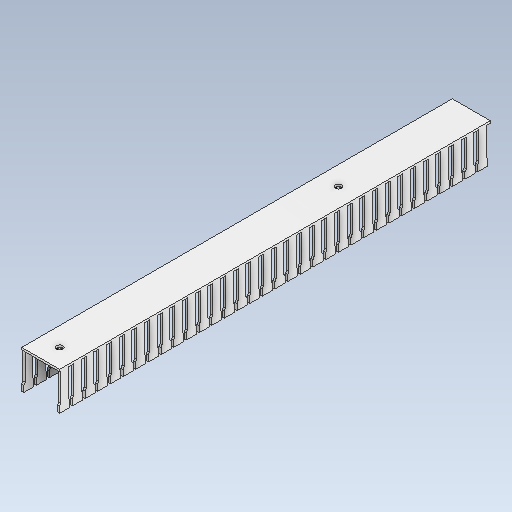
# Autodesk Inventor part: Pasabable Ranurado 30 x 30 L = 430
Saved by Autodesk Inventor 2020 (Build 240168000, 168)
## iProperties
Created: 2020-07-02
Part Number: Pasabable Ranurado 30 x 30 L = 430
Material: PVC-Piping
Document SubType Name: Modeling
Designer: Hernan
Density: 1.4 g/cm^3
Appearance: Smooth - White
Author: Hernan
Autodesk Inventor part; units mm, degrees
ref_plane "YZ Plane" through (0, 0, 0) normal (1, 0, 0) x (0, 1, 0)
ref_plane "XZ Plane" through (0, 0, 0) normal (0, 1, 0) x (-1, 0, 0)
ref_plane "XY Plane" through (0, 0, 0) normal (0, 0, 1) x (1, 0, 0)
sketch "Sketch1" plane through (0, 0, 0) normal (0, 0, 1) x (1, 0, 0)
  line L0 (-26.9918, -9.5406) -> (3.0082, -9.5406)
  line L1 (3.0082, -9.5406) -> (3.0082, 20.4594)
  line L2 (3.0082, 20.4594) -> (-26.9918, 20.4594)
  line L3 (-26.9918, 20.4594) -> (-26.9918, -9.5406)
  line L4 (1.3082, 20.4594) -> (1.3082, -9.5406)
  line L5 (-26.9918, -7.8406) -> (3.0082, -7.8406)
  line L6 (-25.2918, 20.4594) -> (-25.2918, -9.5406)
  line L7 (-26.9918, 18.7594) -> (3.0082, 18.7594)
  point P0 (0, 0)
  point P1 (1.3082, 18.7594)
  point P2 (-25.2918, 18.7594)
  point P3 (-25.2918, -7.8406)
  point P4 (1.3082, -7.8406)
  dimension "d0" = 30
  dimension "d1" = 30
  dimension "d4" = 1.7
  dimension "d5" = 1.7
  dimension "d6" = 1.7
  dimension "d7" = 1.7
  constraints: 16 end point, 8 point on line, 3 horizontal, 3 perpendicular, 2 vertical
  measures "d0" distance of L0.start L0.end
  measures "d1" distance of L0.end L1.end
  measures "d4" distance between parallel lines of L2 L7
  measures "d5" distance between parallel lines of L3 L6
  measures "d6" distance between parallel lines of L0 L5
  measures "d7" distance between parallel lines of L1 L4
extrude "Extrusion1" add sketch "Sketch1" against normal blind 340
extrude "Extrusion2" cut sketch "Sketch1" against normal blind 380 contours L6 L5 L4 L0 | L6 L7 L4 L5
sketch "Boceto2" plane through (-26.9918, 20.4594, 0) normal (0, 1, 0) x (1, 0, 0)
  line L0 (0, 340) -> (30, 340) projected
  line L1 (30, 0) -> (0, 0) projected
  point P0 (26.9918, 0)
sketch "Boceto3" plane through (-26.9918, 20.4594, 0) normal (0, 1, 0) x (1, 0, 0)
  line L0 (28.3, 340) -> (1.7, 340) projected
  line L1 (30, 0) -> (0, 0) projected
  circle A0 centre (15, 235) radius 2.5
  circle A1 centre (15, 15) radius 2.5
  point P0 (26.9918, 0)
  dimension "d17" = 5
  dimension "d18" = 5
  dimension "d95" = 220
  dimension "d97" = 15
  constraints: 2 centre point
  measures "d17" diameter of A0
  measures "d18" diameter of A1
  measures "d95" distance of A1.centre A0.centre
  measures "d97" distance from line of L1 A1.centre
extrude "Extrusión3" cut sketch "Boceto3" against normal blind 10
sketch "Boceto4" plane through (-26.9918, -9.5406, 0) normal (-1, 0, 0) x (0, 0, 1)
  line L0 (0, 0) -> (-8, 0)
  line L1 (0, 0) -> (-340, 0) projected
  line L2 (-8, 0) -> (-8, 5)
  line L3 (-7, 6.5) -> (-7, 28.3)
  line L4 (0, 28.3) -> (-340, 28.3) projected
  line L5 (0, 30) -> (0, 0) projected
  line L6 (0, 0) -> (0, 5)
  line L7 (-1, 6.5) -> (-1, 28.3)
  line L8 (-8, 5) -> (-7, 6.5)
  line L9 (-1, 6.5) -> (0, 5)
  line L10 (-10, 0) -> (-18, 0)
  line L11 (-18, 0) -> (-18, 5)
  line L12 (-17, 6.5) -> (-17, 28.3)
  line L13 (-10, 0) -> (-10, 5)
  line L14 (-11, 6.5) -> (-11, 28.3)
  line L15 (-18, 5) -> (-17, 6.5)
  line L16 (-11, 6.5) -> (-10, 5)
  line L17 (-20, 0) -> (-28, 0)
  line L18 (-28, 0) -> (-28, 5)
  line L19 (-27, 6.5) -> (-27, 28.3)
  line L20 (-20, 0) -> (-20, 5)
  line L21 (-21, 6.5) -> (-21, 28.3)
  line L22 (-28, 5) -> (-27, 6.5)
  line L23 (-21, 6.5) -> (-20, 5)
  line L24 (-30, 0) -> (-38, 0)
  line L25 (-38, 0) -> (-38, 5)
  line L26 (-37, 6.5) -> (-37, 28.3)
  line L27 (-30, 0) -> (-30, 5)
  line L28 (-31, 6.5) -> (-31, 28.3)
  line L29 (-38, 5) -> (-37, 6.5)
  line L30 (-31, 6.5) -> (-30, 5)
  line L31 (-40, 0) -> (-48, 0)
  line L32 (-48, 0) -> (-48, 5)
  line L33 (-47, 6.5) -> (-47, 28.3)
  line L34 (-40, 0) -> (-40, 5)
  line L35 (-41, 6.5) -> (-41, 28.3)
  line L36 (-48, 5) -> (-47, 6.5)
  line L37 (-41, 6.5) -> (-40, 5)
  line L38 (-50, 0) -> (-58, 0)
  line L39 (-58, 0) -> (-58, 5)
  line L40 (-57, 6.5) -> (-57, 28.3)
  line L41 (-50, 0) -> (-50, 5)
  line L42 (-51, 6.5) -> (-51, 28.3)
  line L43 (-58, 5) -> (-57, 6.5)
  line L44 (-51, 6.5) -> (-50, 5)
  line L45 (-60, 0) -> (-68, 0)
  line L46 (-68, 0) -> (-68, 5)
  line L47 (-67, 6.5) -> (-67, 28.3)
  line L48 (-60, 0) -> (-60, 5)
  line L49 (-61, 6.5) -> (-61, 28.3)
  line L50 (-68, 5) -> (-67, 6.5)
  line L51 (-61, 6.5) -> (-60, 5)
  line L52 (-70, 0) -> (-78, 0)
  line L53 (-78, 0) -> (-78, 5)
  line L54 (-77, 6.5) -> (-77, 28.3)
  line L55 (-70, 0) -> (-70, 5)
  line L56 (-71, 6.5) -> (-71, 28.3)
  line L57 (-78, 5) -> (-77, 6.5)
  line L58 (-71, 6.5) -> (-70, 5)
  line L59 (-80, 0) -> (-88, 0)
  line L60 (-88, 0) -> (-88, 5)
  line L61 (-87, 6.5) -> (-87, 28.3)
  line L62 (-80, 0) -> (-80, 5)
  line L63 (-81, 6.5) -> (-81, 28.3)
  line L64 (-88, 5) -> (-87, 6.5)
  line L65 (-81, 6.5) -> (-80, 5)
  line L66 (-90, 0) -> (-98, 0)
  line L67 (-98, 0) -> (-98, 5)
  line L68 (-97, 6.5) -> (-97, 28.3)
  line L69 (-90, 0) -> (-90, 5)
  line L70 (-91, 6.5) -> (-91, 28.3)
  line L71 (-98, 5) -> (-97, 6.5)
  line L72 (-91, 6.5) -> (-90, 5)
  line L73 (-100, 0) -> (-108, 0)
  line L74 (-108, 0) -> (-108, 5)
  line L75 (-107, 6.5) -> (-107, 28.3)
  line L76 (-100, 0) -> (-100, 5)
  line L77 (-101, 6.5) -> (-101, 28.3)
  line L78 (-108, 5) -> (-107, 6.5)
  line L79 (-101, 6.5) -> (-100, 5)
  line L80 (-110, 0) -> (-118, 0)
  line L81 (-118, 0) -> (-118, 5)
  line L82 (-117, 6.5) -> (-117, 28.3)
  line L83 (-110, 0) -> (-110, 5)
  line L84 (-111, 6.5) -> (-111, 28.3)
  line L85 (-118, 5) -> (-117, 6.5)
  line L86 (-111, 6.5) -> (-110, 5)
  line L87 (-120, 0) -> (-128, 0)
  line L88 (-128, 0) -> (-128, 5)
  line L89 (-127, 6.5) -> (-127, 28.3)
  line L90 (-120, 0) -> (-120, 5)
  line L91 (-121, 6.5) -> (-121, 28.3)
  line L92 (-128, 5) -> (-127, 6.5)
  line L93 (-121, 6.5) -> (-120, 5)
  line L94 (-130, 0) -> (-138, 0)
  line L95 (-138, 0) -> (-138, 5)
  line L96 (-137, 6.5) -> (-137, 28.3)
  line L97 (-130, 0) -> (-130, 5)
  line L98 (-131, 6.5) -> (-131, 28.3)
  line L99 (-138, 5) -> (-137, 6.5)
  line L100 (-131, 6.5) -> (-130, 5)
  line L101 (-140, 0) -> (-148, 0)
  line L102 (-148, 0) -> (-148, 5)
  line L103 (-147, 6.5) -> (-147, 28.3)
  line L104 (-140, 0) -> (-140, 5)
  line L105 (-141, 6.5) -> (-141, 28.3)
  line L106 (-148, 5) -> (-147, 6.5)
  line L107 (-141, 6.5) -> (-140, 5)
  line L108 (-150, 0) -> (-158, 0)
  line L109 (-158, 0) -> (-158, 5)
  line L110 (-157, 6.5) -> (-157, 28.3)
  line L111 (-150, 0) -> (-150, 5)
  line L112 (-151, 6.5) -> (-151, 28.3)
  line L113 (-158, 5) -> (-157, 6.5)
  line L114 (-151, 6.5) -> (-150, 5)
  line L115 (-160, 0) -> (-168, 0)
  line L116 (-168, 0) -> (-168, 5)
  line L117 (-167, 6.5) -> (-167, 28.3)
  line L118 (-160, 0) -> (-160, 5)
  line L119 (-161, 6.5) -> (-161, 28.3)
  line L120 (-168, 5) -> (-167, 6.5)
  line L121 (-161, 6.5) -> (-160, 5)
  line L122 (-170, 0) -> (-178, 0)
  line L123 (-178, 0) -> (-178, 5)
  line L124 (-177, 6.5) -> (-177, 28.3)
  line L125 (-170, 0) -> (-170, 5)
  line L126 (-171, 6.5) -> (-171, 28.3)
  line L127 (-178, 5) -> (-177, 6.5)
  line L128 (-171, 6.5) -> (-170, 5)
  line L129 (-180, 0) -> (-188, 0)
  line L130 (-188, 0) -> (-188, 5)
  line L131 (-187, 6.5) -> (-187, 28.3)
  line L132 (-180, 0) -> (-180, 5)
  line L133 (-181, 6.5) -> (-181, 28.3)
  line L134 (-188, 5) -> (-187, 6.5)
  line L135 (-181, 6.5) -> (-180, 5)
  line L136 (-190, 0) -> (-198, 0)
  line L137 (-198, 0) -> (-198, 5)
  line L138 (-197, 6.5) -> (-197, 28.3)
  line L139 (-190, 0) -> (-190, 5)
  line L140 (-191, 6.5) -> (-191, 28.3)
  line L141 (-198, 5) -> (-197, 6.5)
  line L142 (-191, 6.5) -> (-190, 5)
  line L143 (-200, 0) -> (-208, 0)
  line L144 (-208, 0) -> (-208, 5)
  line L145 (-207, 6.5) -> (-207, 28.3)
  line L146 (-200, 0) -> (-200, 5)
  line L147 (-201, 6.5) -> (-201, 28.3)
  line L148 (-208, 5) -> (-207, 6.5)
  line L149 (-201, 6.5) -> (-200, 5)
  line L150 (-210, 0) -> (-218, 0)
  line L151 (-218, 0) -> (-218, 5)
  line L152 (-217, 6.5) -> (-217, 28.3)
  line L153 (-210, 0) -> (-210, 5)
  line L154 (-211, 6.5) -> (-211, 28.3)
  line L155 (-218, 5) -> (-217, 6.5)
  line L156 (-211, 6.5) -> (-210, 5)
  line L157 (-220, 0) -> (-228, 0)
  line L158 (-228, 0) -> (-228, 5)
  line L159 (-227, 6.5) -> (-227, 28.3)
  line L160 (-220, 0) -> (-220, 5)
  line L161 (-221, 6.5) -> (-221, 28.3)
  line L162 (-228, 5) -> (-227, 6.5)
  line L163 (-221, 6.5) -> (-220, 5)
  line L164 (-230, 0) -> (-238, 0)
  line L165 (-238, 0) -> (-238, 5)
  line L166 (-237, 6.5) -> (-237, 28.3)
  line L167 (-230, 0) -> (-230, 5)
  line L168 (-231, 6.5) -> (-231, 28.3)
  line L169 (-238, 5) -> (-237, 6.5)
  line L170 (-231, 6.5) -> (-230, 5)
  line L171 (-240, 0) -> (-248, 0)
  line L172 (-248, 0) -> (-248, 5)
  line L173 (-247, 6.5) -> (-247, 28.3)
  line L174 (-240, 0) -> (-240, 5)
  line L175 (-241, 6.5) -> (-241, 28.3)
  line L176 (-248, 5) -> (-247, 6.5)
  line L177 (-241, 6.5) -> (-240, 5)
  line L178 (-250, 0) -> (-258, 0)
  line L179 (-258, 0) -> (-258, 5)
  line L180 (-257, 6.5) -> (-257, 28.3)
  line L181 (-250, 0) -> (-250, 5)
  line L182 (-251, 6.5) -> (-251, 28.3)
  line L183 (-258, 5) -> (-257, 6.5)
  line L184 (-251, 6.5) -> (-250, 5)
  line L185 (-260, 0) -> (-268, 0)
  line L186 (-268, 0) -> (-268, 5)
  line L187 (-267, 6.5) -> (-267, 28.3)
  line L188 (-260, 0) -> (-260, 5)
  line L189 (-261, 6.5) -> (-261, 28.3)
  line L190 (-268, 5) -> (-267, 6.5)
  line L191 (-261, 6.5) -> (-260, 5)
  line L192 (-270, 0) -> (-278, 0)
  line L193 (-278, 0) -> (-278, 5)
  line L194 (-277, 6.5) -> (-277, 28.3)
  line L195 (-270, 0) -> (-270, 5)
  line L196 (-271, 6.5) -> (-271, 28.3)
  line L197 (-278, 5) -> (-277, 6.5)
  line L198 (-271, 6.5) -> (-270, 5)
  line L199 (-280, 0) -> (-288, 0)
  line L200 (-288, 0) -> (-288, 5)
  line L201 (-287, 6.5) -> (-287, 28.3)
  line L202 (-280, 0) -> (-280, 5)
  line L203 (-281, 6.5) -> (-281, 28.3)
  line L204 (-288, 5) -> (-287, 6.5)
  line L205 (-281, 6.5) -> (-280, 5)
  line L206 (0, 28.3) -> (-340, 28.3)
  line L207 (0, 30) -> (-340, 30) projected
  line L208 (0, 30) -> (0, 5)
  line L209 (-290, 0) -> (-290, 5)
  line L210 (-290, 0) -> (-298, 0)
  line L211 (-298, 0) -> (-298, 5)
  line L212 (-297, 6.5) -> (-297, 28.3)
  line L213 (-291, 6.5) -> (-291, 28.3)
  line L214 (-298, 5) -> (-297, 6.5)
  line L215 (-291, 6.5) -> (-290, 5)
  line L216 (-300, 0) -> (-300, 5)
  line L217 (-300, 0) -> (-308, 0)
  line L218 (-308, 0) -> (-308, 5)
  line L219 (-307, 6.5) -> (-307, 28.3)
  line L220 (-301, 6.5) -> (-301, 28.3)
  line L221 (-308, 5) -> (-307, 6.5)
  line L222 (-301, 6.5) -> (-300, 5)
  line L223 (-310, 0) -> (-310, 5)
  line L224 (-310, 0) -> (-318, 0)
  line L225 (-318, 0) -> (-318, 5)
  line L226 (-317, 6.5) -> (-317, 28.3)
  line L227 (-311, 6.5) -> (-311, 28.3)
  line L228 (-318, 5) -> (-317, 6.5)
  line L229 (-311, 6.5) -> (-310, 5)
  line L230 (-320, 0) -> (-320, 5)
  line L231 (-320, 0) -> (-328, 0)
  line L232 (-328, 0) -> (-328, 5)
  line L233 (-327, 6.5) -> (-327, 28.3)
  line L234 (-321, 6.5) -> (-321, 28.3)
  line L235 (-328, 5) -> (-327, 6.5)
  line L236 (-321, 6.5) -> (-320, 5)
  line L237 (-330, 0) -> (-330, 5)
  line L238 (-330, 0) -> (-338, 0)
  line L239 (-338, 0) -> (-338, 5)
  line L240 (-337, 6.5) -> (-337, 28.3)
  line L241 (-331, 6.5) -> (-331, 28.3)
  line L242 (-338, 5) -> (-337, 6.5)
  line L243 (-331, 6.5) -> (-330, 5)
  line L244 (-338, 0) -> (-340, 0)
  line L245 (-340, 0) -> (-340, 28.3)
  line L246 (-340, 30) -> (-340, 0) projected
  point P0 (0, 9.5406)
  point P1 (-338, 0)
  point P2 (-330, 0)
  point P3 (-328, 0)
  point P4 (-320, 0)
  point P5 (-318, 0)
  point P6 (-310, 0)
  point P7 (-287, 28.3)
  point P8 (-267, 28.3)
  point P9 (-261, 28.3)
  point P10 (-251, 28.3)
  point P11 (-241, 28.3)
  point P12 (-231, 28.3)
  point P13 (-221, 28.3)
  point P14 (-211, 28.3)
  point P15 (-201, 28.3)
  point P16 (-121, 28.3)
  point P17 (-111, 28.3)
  point P18 (-101, 28.3)
  point P19 (-91, 28.3)
  dimension "d21" = 8
  dimension "d26" = 8
  dimension "d27" = 8
  dimension "d28" = 8
  dimension "d29" = 8
  dimension "d30" = 8
  dimension "d31" = 8
  dimension "d32" = 8
  dimension "d33" = 8
  dimension "d34" = 8
  dimension "d35" = 8
  dimension "d36" = 8
  dimension "d37" = 8
  dimension "d38" = 8
  dimension "d39" = 8
  dimension "d40" = 8
  dimension "d41" = 8
  dimension "d42" = 8
  dimension "d43" = 8
  dimension "d44" = 8
  dimension "d45" = 8
  dimension "d46" = 8
  dimension "d47" = 8
  dimension "d48" = 8
  dimension "d49" = 8
  dimension "d50" = 8
  dimension "d51" = 8
  dimension "d52" = 8
  dimension "d53" = 8
  dimension "d55" = 2
  dimension "d56" = 2
  dimension "d57" = 2
  dimension "d58" = 2
  dimension "d59" = 2
  dimension "d60" = 2
  dimension "d61" = 2
  dimension "d62" = 2
  dimension "d63" = 2
  dimension "d64" = 2
  dimension "d65" = 2
  dimension "d66" = 2
  dimension "d67" = 2
  dimension "d68" = 2
  dimension "d69" = 2
  dimension "d70" = 2
  dimension "d71" = 2
  dimension "d72" = 2
  dimension "d73" = 2
  dimension "d74" = 2
  dimension "d75" = 2
  dimension "d76" = 2
  dimension "d77" = 2
  dimension "d78" = 2
  dimension "d79" = 2
  dimension "d80" = 2
  dimension "d81" = 2
  dimension "d82" = 2
  dimension "d83" = 8
  dimension "d84" = 8
  dimension "d85" = 8
  dimension "d86" = 8
  dimension "d87" = 8
  dimension "d88" = 2
  dimension "d89" = 2
  constraints: 484 end point, 35 perpendicular, 2 horizontal, 1 collinear, 4 other
  measures "d21" distance of L0.start L0.end
  measures "d26" distance of L13.start L10.end
  measures "d27" distance of L20.start L17.end
  measures "d28" distance of L27.start L24.end
  measures "d29" distance of L34.start L31.end
  measures "d30" distance of L41.start L38.end
  measures "d31" distance of L48.start L45.end
  measures "d32" distance of L55.start L52.end
  measures "d33" distance of L62.start L59.end
  measures "d34" distance of L69.start L66.end
  measures "d35" distance of L76.start L73.end
  measures "d36" distance of L83.start L80.end
  measures "d37" distance of L90.start L87.end
  measures "d38" distance of L97.start L94.end
  measures "d39" distance of L104.start L101.end
  measures "d40" distance of L111.start L108.end
  measures "d41" distance of L118.start L115.end
  measures "d42" distance of L125.start L122.end
  measures "d43" distance of L132.start L129.end
  measures "d44" distance of L139.start L136.end
  measures "d45" distance of L146.start L143.end
  measures "d46" distance of L153.start L150.end
  measures "d47" distance of L160.start L157.end
  measures "d48" distance of L167.start L164.end
  measures "d49" distance of L174.start L171.end
  measures "d50" distance of L181.start L178.end
  measures "d51" distance of L188.start L185.end
  measures "d52" distance of L195.start L192.end
  measures "d53" distance of L202.start L199.end
  measures "d55" distance of L13.start L0.end
  measures "d56" distance of L20.start L10.end
  measures "d57" distance of L27.start L17.end
  measures "d58" distance of L34.start L24.end
  measures "d59" distance of L41.start L31.end
  measures "d60" distance of L48.start L38.end
  measures "d61" distance of L55.start L45.end
  measures "d62" distance of L62.start L52.end
  measures "d63" distance of L69.start L59.end
  measures "d64" distance of L76.start L66.end
  measures "d65" distance of L83.start L73.end
  measures "d66" distance of L90.start L80.end
  measures "d67" distance of L97.start L87.end
  measures "d68" distance of L104.start L94.end
  measures "d69" distance of L111.start L101.end
  measures "d70" distance of L118.start L108.end
  measures "d71" distance of L125.start L115.end
  measures "d72" distance of L132.start L122.end
  measures "d73" distance of L139.start L129.end
  measures "d74" distance of L146.start L136.end
  measures "d75" distance of L153.start L143.end
  measures "d76" distance of L160.start L150.end
  measures "d77" distance of L167.start L157.end
  measures "d78" distance of L174.start L164.end
  measures "d79" distance of L181.start L171.end
  measures "d80" distance of L188.start L178.end
  measures "d81" distance of L195.start L185.end
  measures "d82" distance of L202.start L192.end
  measures "d83" distance of L210.start L210.end
  measures "d84" distance of L217.start L217.end
  measures "d85" distance of L224.start L224.end
  measures "d86" distance of L231.start L231.end
  measures "d87" distance of L238.start L238.end
  measures "d88" distance of L210.start L199.end
  measures "d89" distance of L217.start L210.end
extrude "Extrusión4" cut sketch "Boceto4" against normal blind 30 contours L1 L13 L16 L14 L4 L3 L8 L2 | L9 L7 L4 L5 | L1 L20 L23 L21 L4 L12 L15 L11 | L1 L27 L30 L28 L4 L19 L22 L18 | L4 L240 L242 L239 L1 L245 | L1 L34 L37 L35 L4 L26 L29 L25 | L4 L233 L235 L232 L1 L237 L243 L241 | L1 L41 L44 L42 L4 L33 L36 L32 | L4 L226 L228 L225 L1 L230 L236 L234 | L1 L48 L51 L49 L4 L40 L43 L39 | L4 L219 L221 L218 L1 L223 L229 L227 | L1 L55 L58 L56 L4 L47 L50 L46 | L4 L212 L214 L211 L1 L216 L222 L220 | L1 L62 L65 L63 L4 L54 L57 L53 | L4 L201 L204 L200 L1 L209 L215 L213 | L1 L69 L72 L70 L4 L61 L64 L60 | L4 L194 L197 L193 L1 L202 L205 L203 | L1 L76 L79 L77 L4 L68 L71 L67 | L4 L187 L190 L186 L1 L195 L198 L196 | L1 L83 L86 L84 L4 L75 L78 L74 | L4 L180 L183 L179 L1 L188 L191 L189 | L1 L90 L93 L91 L4 L82 L85 L81 | L4 L173 L176 L172 L1 L181 L184 L182 | L1 L97 L100 L98 L4 L89 L92 L88 | L4 L166 L169 L165 L1 L174 L177 L175 | L1 L104 L107 L105 L4 L96 L99 L95 | L4 L159 L162 L158 L1 L167 L170 L168 | L1 L111 L114 L112 L4 L103 L106 L102 | L4 L152 L155 L151 L1 L160 L163 L161 | L1 L118 L121 L119 L4 L110 L113 L109 | L4 L145 L148 L144 L1 L153 L156 L154 | L1 L125 L128 L126 L4 L117 L120 L116 | L4 L138 L141 L137 L1 L146 L149 L147 | L1 L132 L135 L133 L4 L124 L127 L123 | L4 L131 L134 L130 L1 L139 L142 L140
body "Solid1"
